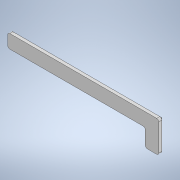
# Autodesk Inventor part: Z Alignment Guide
Saved by Autodesk Inventor 2022 (Build 260153000, 153)
## iProperties
Created: 2022-02-22
Part Number: Z Alignment Guide
Material: Generic
Document SubType Name: Modeling
Designer: nicol
Density: 1 g/cm^3
Appearance: Default
Author: nicol
Autodesk Inventor part; units mm, degrees
ref_plane "YZ Plane" through (0, 0, 0) normal (1, 0, 0) x (0, 1, 0)
ref_plane "XZ Plane" through (0, 0, 0) normal (0, 1, 0) x (-1, 0, 0)
ref_plane "XY Plane" through (0, 0, 0) normal (0, 0, 1) x (1, 0, 0)
sketch "Sketch1" plane through (0, 0, 0) normal (0, 0, 1) x (1, 0, 0)
  line L0 (0, 0) -> (132.5, 0)
  line L1 (132.5, 0) -> (132.5, 10)
  line L2 (132.5, 10) -> (0, 10)
  line L3 (0, 10) -> (0, 0)
  line L4 (132.5, 0) -> (132.5, -20)
  line L5 (132.5, -20) -> (142.5, -20)
  line L6 (142.5, -20) -> (142.5, 10)
  line L7 (142.5, 10) -> (132.5, 10)
  line L8 (0, 0) -> (0, -3)
  line L9 (0, -3) -> (129.5, -3)
  line L10 (129.5, -3) -> (129.5, -20)
  line L11 (129.5, -20) -> (132.5, -20)
  dimension "d0" = 132.5
  dimension "d1" = 10
  dimension "d2" = 10
  dimension "d3" = 20
  dimension "d4" = 3
  dimension "d5" = 3
  constraints: 24 end point, 5 perpendicular, 3 vertical, 2 horizontal, 2 parallel
  measures "d0" distance of L2.end L1.end
  measures "d1" distance of L1.end L0.end
  measures "d2" distance of L6.end L1.end
  measures "d3" distance of L0.end L4.end
  measures "d4" distance between parallel lines of L0 L9
  measures "d5" distance between parallel lines of L4 L10
extrude "Extrusion1" add sketch "Sketch1" along normal blind 3
extrude "Extrusion2" add sketch "Sketch1" against normal blind 10 contours L0 L4 L11 L10 L9 L8
sketch "Sketch2" plane through (0, -3, 3) normal (-1, 0, 0) x (0, 0, 1)
  line L0 (-13, 3) -> (-13, -17) projected
  line L1 (-13, 3) -> (-3, 12.9668)
  line L2 (-3, 13) -> (-3, 3) projected
  line L3 (-3, 3) -> (-13, 3) projected
  line L4 (-13, 0) -> (-13, 3) projected
  line L5 (-13, 0) -> (0, 0) projected
  line L6 (0, 13) -> (0, 0) projected
  line L7 (-3, 13) -> (0, 13) projected
  constraints: 2 end point
extrude "Extrusion3" add sketch "Sketch2" along normal blind 3
fillet "Fillet2" radius 2 6 edges at (142.5, 10, 1.5) (142.5, -20, 1.5) (129.5, -20, -3.5) (129.5, -3, -3.5) (-3, 10, 1.5) (-3, -3, -3.5)
body "Solid1"
